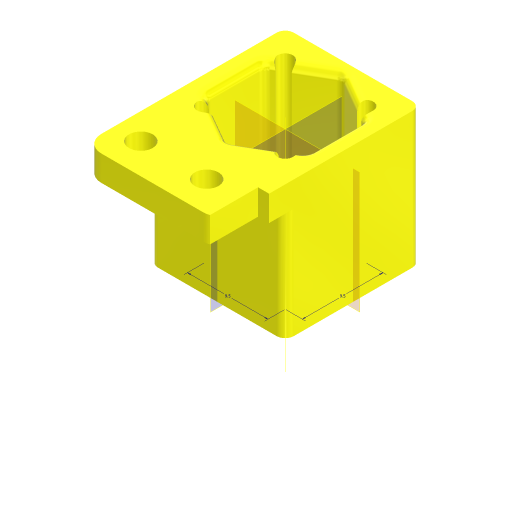
# Autodesk Inventor part: 30_Laser_to_M12Adapter_9,5mm
Saved by Autodesk Inventor 2024.1 (Build 281209000, 209)
## iProperties
Created: 2023-02-07
Part Number: 30_Laser_to_M12Adapter_9,5mm
Material: Generisch
Document SubType Name: Modeling
Designer: diederichbenedict
Density: 1 g/cm^3
Appearance: Glatt - Gelb
Author: diederichbenedict
Autodesk Inventor part; units mm, degrees
ref_plane "YZ Plane" through (0, 0, 0) normal (1, 0, 0) x (0, 1, 0)
ref_plane "XZ Plane" through (0, 0, 0) normal (0, 1, 0) x (-1, 0, 0)
ref_plane "XY Plane" through (0, 0, 0) normal (0, 0, 1) x (1, 0, 0)
sketch "Skizze1" plane through (0, 0, 0) normal (0, 1, 0) x (-1, 0, 0)
  line L0 (-8, -8) -> (8, -8)
  line L1 (8, -8) -> (8, 8)
  line L2 (8, 8) -> (-8, 8)
  line L3 (-8, 8) -> (-8, -8)
  line L4 (-8, -8) -> (8, 8) construction
  line L5 (8, -8) -> (-8, 8) construction
  circle A0 centre (0, 0) radius 3
  line L6 (4.75, -4.75) -> (-4.75, -4.75) construction
  line L7 (-4.75, -4.75) -> (-4.75, 4.75) construction
  line L8 (-4.75, 4.75) -> (4.75, 4.75) construction
  line L9 (4.75, 4.75) -> (4.75, -4.75) construction
  line L10 (4.75, -4.75) -> (-4.75, 4.75) construction
  line L11 (-4.75, -4.75) -> (4.75, 4.75) construction
  circle A1 centre (-4.75, 4.75) radius 0.9
  circle A2 centre (-4.75, -4.75) radius 0.9
  circle A3 centre (4.75, -4.75) radius 0.9
  circle A4 centre (4.75, 4.75) radius 0.9
  dimension "d0" = 16
  dimension "d1" = 16
  dimension "d21" = 6
  dimension "d22" = 9.5
  dimension "d23" = 9.5
  dimension "d24" = 1.8
  dimension "d25" = 1.8
  dimension "d26" = 1.8
  dimension "d27" = 1.8
  constraints: 24 end point, 6 coincident, 5 centre point, 4 midpoint, 4 parallel, 2 horizontal, 2 perpendicular
  measures "d0" distance of L2.end L1.end
  measures "d1" distance of L1.end L0.end
  measures "d21" diameter of A0
  measures "d22" distance of L7.end L8.end
  measures "d23" distance of L6.end L7.end
  measures "d24" diameter of A1
  measures "d25" diameter of A2
  measures "d26" diameter of A3
  measures "d27" diameter of A4
extrude "Extrusion1" add sketch "Skizze1" along normal blind 3
fillet "Rundung1" [suppressed]
sketch "Skizze2" plane through (0, 3, 0) normal (0, 1, 0) x (1, 0, 0)
  line L0 (-8, 8) -> (-8, -8) projected
  line L1 (-8, -8) -> (8, -8) projected
  line L2 (8, -8) -> (8, 8) projected
  line L3 (8, 8) -> (-8, 8) projected
  line L4 (0, -6.8416) -> (-5.925, -3.4208)
  line L5 (-5.925, -3.4208) -> (-5.925, 3.4208)
  line L6 (-5.925, 3.4208) -> (0, 6.8416)
  line L7 (0, 6.8416) -> (5.925, 3.4208)
  line L8 (5.925, 3.4208) -> (5.925, -3.4208)
  line L9 (5.925, -3.4208) -> (0, -6.8416)
  line L10 (-8, 8) -> (-8, -8) projected
  line L11 (8, 8) -> (-8, 8) projected
  line L12 (8, -8) -> (8, 8) projected
  line L13 (-8, -8) -> (8, -8) projected
  circle A0 centre (0, 0) radius 3 projected
  circle A1 centre (4.75, -4.75) radius 0.9 projected
  circle A2 centre (4.75, 4.75) radius 0.9 projected
  circle A3 centre (-4.75, 4.75) radius 0.9 projected
  circle A4 centre (-4.75, -4.75) radius 0.9 projected
  point P0 (8, 5.7735)
  point P1 (8, -5.7735)
  point P2 (-8, -5.7735)
  point P3 (-8, 5.7735)
  point P4 (4.1436, -8)
  point P5 (-4.1436, -8)
  point P6 (4.1436, 8)
  point P7 (-4.1436, 8)
  point P8 (-5.0758, 3.9111)
  point P9 (-3.8605, 4.6127)
  point P10 (3.8605, 4.6127)
  point P11 (5.0758, 3.9111)
  point P12 (5.0758, -3.9111)
  point P13 (3.8605, -4.6127)
  point P14 (-3.8605, -4.6127)
  point P15 (-5.0758, -3.9111)
  dimension "d6" = 11.85
  constraints: 12 end point, 1 coincident, 13 other
  measures "d6" distance between parallel lines of L8 L5
extrude "Extrusion2" add sketch "Skizze2" along normal blind 13 contours L3 L2 L1 L0
fillet "Rundung2" radius 1 20 edges at (0, 9.5, 6.8416) (-5.925, 9.5, 3.4208) (-5.925, 9.5, -3.4208) (0, 9.5, -6.8416) (5.925, 9.5, -3.4208) (5.925, 9.5, 3.4208) (8, 8, -8) (-8, 8, -8) (-8, 8, 8) (8, 8, 8) (-5.5004, 16, -3.6659) (-1.9303, 16, -5.7272) (-5.925, 16, 0) (-1.9303, 16, 5.7272) (-5.5004, 16, 3.6659) (5.5004, 16, 3.6659) (1.9303, 16, 5.7272) (5.925, 16, 0) (1.9303, 16, -5.7272) (5.5004, 16, -3.6659)
ref_plane "Arbeitsebene1" through (0, 0, -8) normal (-1, 0, 0) x (0, 0, 1)
ref_plane "Arbeitsebene2" through (-8, 0, 0) normal (0, 0, 1) x (1, 0, 0)
sketch "Skizze3" plane through (0, 16, 0) normal (0, 1, 0) x (1, 0, 0)
  arc A0 (7, -8) -> (8, -7) centre (7, -7) ccw projected
  line L0 (8, -7) -> (8, 7) projected
  arc A1 (8, 7) -> (7, 8) centre (7, 7) ccw projected
  line L1 (7, 8) -> (-7, 8) projected
  arc A2 (-7, 8) -> (-8, 7) centre (-7, 7) ccw projected
  line L2 (-8, 7) -> (-8, -7) projected
  arc A3 (-8, -7) -> (-7, -8) centre (-7, -7) ccw projected
  line L3 (-7, -8) -> (7, -8) projected
  arc A4 (-1, -7.419) -> (1, -7.419) centre (0, -5.6869) ccw projected
  line L4 (-4.2865, -5.5215) -> (-1, -7.419) projected
  arc A5 (-6.925, -2.8435) -> (-5.925, -4.5755) centre (-4.925, -2.8435) ccw projected
  line L5 (-6.925, 2.8435) -> (-6.925, -2.8435) projected
  arc A6 (-5.925, 4.5755) -> (-6.925, 2.8435) centre (-4.925, 2.8435) ccw projected
  line L6 (-5.6499, 4.7344) -> (-5.925, 4.5755) projected
  arc A7 (1, 7.419) -> (-1, 7.419) centre (0, 5.6869) ccw projected
  line L7 (5.925, 4.5755) -> (5.6499, 4.7344) projected
  arc A8 (6.925, 2.8435) -> (5.925, 4.5755) centre (4.925, 2.8435) ccw projected
  line L8 (6.925, -2.8435) -> (6.925, 2.8435) projected
  arc A9 (5.925, -4.5755) -> (6.925, -2.8435) centre (4.925, -2.8435) ccw projected
  line L9 (5.6499, -4.7344) -> (5.925, -4.5755) projected
  line L10 (-8, -5.6869) -> (8, -5.6869)
  line L11 (8, -5.6869) -> (8, -13.6869)
  line L12 (6, -15.6869) -> (-6, -15.6869)
  line L13 (-8, -13.6869) -> (-8, -5.6869)
  circle A10 centre (-4.925, -12.0977) radius 1.4
  circle A11 centre (2.836, -12.0977) radius 1.4
  arc A12 (-8, -13.6869) -> (-6, -15.6869) centre (-6, -13.6869) ccw
  arc A13 (6, -15.6869) -> (8, -13.6869) centre (6, -13.6869) ccw
  arc A14 (4.2865, -5.5215) -> (5.6499, -4.7344) centre (4.75, -4.75) ccw projected
  line L14 (1, -7.419) -> (4.2865, -5.5215) projected
  arc A15 (-5.6499, -4.7344) -> (-4.2865, -5.5215) centre (-4.75, -4.75) ccw projected
  line L15 (-5.925, -4.5755) -> (-5.6499, -4.7344) projected
  arc A16 (-4.2865, 5.5215) -> (-5.6499, 4.7344) centre (-4.75, 4.75) ccw projected
  line L16 (-1, 7.419) -> (-4.2865, 5.5215) projected
  line L17 (4.2865, 5.5215) -> (1, 7.419) projected
  arc A17 (5.6499, 4.7344) -> (4.2865, 5.5215) centre (4.75, 4.75) ccw projected
  point P0 (0, 0)
  point P1 (8, -15.6869)
  point P2 (8, -7)
  dimension "d10" = 10
  dimension "d11" = 2.8
  dimension "d12" = 2.8
  dimension "d13" = 2
  constraints: 8 end point, 4 centre point, 4 point on circle, 4 tangent, 3 point on line, 2 parallel, 1 equal radius, 1 horizontal, 1 perpendicular
  measures "d10" distance of L10.end point (8, -15.687)
  measures "d11" diameter of A10
  measures "d12" diameter of A11
  measures "d13" radius of A12
extrude "Extrusion3" add sketch "Skizze3" against normal blind 3 contours A0 L11 A13 L12 A12 L13 A3 L3
sketch "Skizze4" plane through (0, 0, 0) normal (0, -1, 0) x (1, 0, 0)
  line L0 (12.8, 30) -> (12.8, 10) projected
  line L1 (12.8, 30) -> (6.8, 30) projected
  line L2 (6.8, 10) -> (6.8, 30) projected
  line L3 (12.8, 10) -> (6.8, 10) projected
  line L4 (6.7, 30.1) -> (12.9, 30.1)
  line L5 (12.9, 30.1) -> (12.9, 9.9)
  line L6 (12.9, 9.9) -> (6.7, 9.9)
  line L7 (6.7, 9.9) -> (6.7, 30.1)
  point P0 (0, 0)
  dimension "d16" = 0.1
  constraints: 8 end point, 3 other
  measures "d16" distance between parallel lines of L2 L7
extrude "Extrusion4" cut sketch "Skizze4" against normal through all contours L0 L3 L2 L1 | L4 L5 L6 L7
sketch "Skizze5" plane through (0, 0, 0) normal (0, -1, 0) x (1, 0, 0)
  line L0 (-4.75, -4.75) -> (4.75, -4.75)
  line L1 (4.75, -4.75) -> (4.75, 4.75)
  line L2 (4.75, 4.75) -> (-4.75, 4.75)
  line L3 (-4.75, 4.75) -> (-4.75, -4.75)
  line L4 (-4.75, -4.75) -> (4.75, 4.75) construction
  line L5 (4.75, -4.75) -> (-4.75, 4.75) construction
  point P0 (0, 0)
  dimension "d19" = 9.5
  dimension "d20" = 9.5
  constraints: 12 end point, 2 midpoint, 2 parallel, 1 horizontal, 1 perpendicular
  measures "d19" distance of L2.end L1.end
  measures "d20" distance of L1.end L0.end
